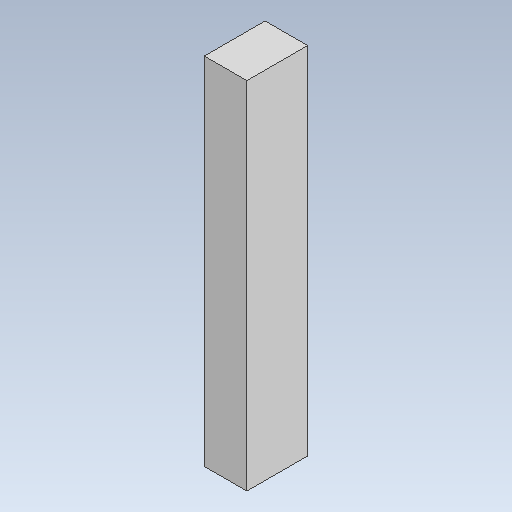
# Autodesk Inventor part: right stem
Saved by Autodesk Inventor 2021 (Build 250183000, 183)
## iProperties
Created: 2021-06-25
Part Number: right stem
Material: Generic
Document SubType Name: Modeling
Designer: TARUN
Density: 1 g/cm^3
Appearance: Default
Author: TARUN
Autodesk Inventor part; units mm, degrees
ref_plane "YZ Plane" through (0, 0, 0) normal (1, 0, 0) x (0, 1, 0)
ref_plane "XZ Plane" through (0, 0, 0) normal (0, 1, 0) x (-1, 0, 0)
ref_plane "XY Plane" through (0, 0, 0) normal (0, 0, 1) x (1, 0, 0)
sketch "Sketch2" plane through (0, 0, 0) normal (0, 1, 0) x (-1, 0, 0)
  line L0 (-0.3507, -1.9885) -> (-7.3507, -1.9885)
  line L1 (-7.3507, -1.9885) -> (-7.3507, 8.0115)
  line L2 (-7.3507, 8.0115) -> (-0.3507, 8.0115)
  line L3 (-0.3507, 8.0115) -> (-0.3507, -1.9885)
  point P0 (0, 0)
  dimension "d2" = 7
  dimension "d3" = 10
  constraints: 8 end point, 2 parallel, 1 horizontal, 1 perpendicular
  measures "d2" distance of L1.end L2.end
  measures "d3" distance of L0.end L1.end
extrude "Extrusion1" add sketch "Sketch2" along normal blind 58.493
body "Solid1"
